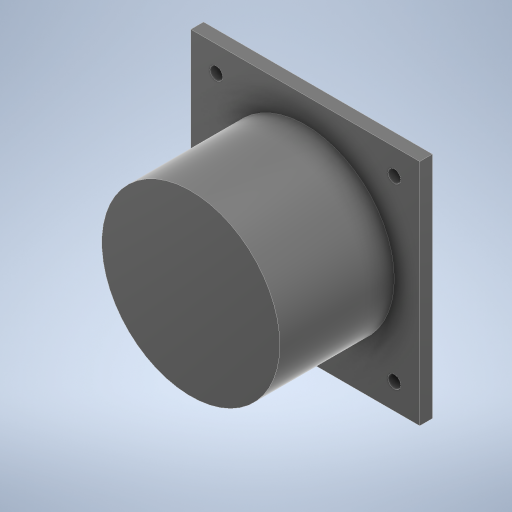
# Autodesk Inventor part: Steckdose
Saved by Autodesk Inventor 2024 (Build 280153000, 153)
## iProperties
Created: 2026-06-01
Part Number: Steckdose
Material: PC/ABS-Kunststoff
Document SubType Name: Modeling
Designer: maxim
Density: 1.1 g/cm^3
Appearance: Glatt - Schwarz
Author: maxim
Autodesk Inventor part; units mm, degrees
ref_plane "YZ Plane" through (0, 0, 0) normal (1, 0, 0) x (0, 1, 0)
ref_plane "XZ Plane" through (0, 0, 0) normal (0, 1, 0) x (-1, 0, 0)
ref_plane "XY Plane" through (0, 0, 0) normal (0, 0, 1) x (1, 0, 0)
sketch "Skizze1" plane through (0, 0, 0) normal (0, 1, 0) x (-1, 0, 0)
  line L0 (0, 0) -> (72, 0)
  line L1 (72, 0) -> (72, -72)
  line L2 (72, -72) -> (0, -72)
  line L3 (0, -72) -> (0, 0)
  dimension "d6" = 72
  dimension "STECKDOSE" = 72
  constraints: 8 end point, 2 parallel, 1 horizontal, 1 perpendicular
  measures "d6" distance of L1.end L2.end
  measures "STECKDOSE" distance of L0.end L1.end
extrude "Extrusion1" add sketch "Skizze1" along normal blind 5
sketch "Skizze2" plane through (0, 5, 0) normal (0, 1, 0) x (1, 0, 0)
  line L0 (-72, 72) -> (-72, 0) projected
  line L1 (0, 0) -> (0, 72) projected
  line L2 (-72, 0) -> (0, 0) projected
  point P0 (-8, 8)
  dimension "d23" = 8
  dimension "d24" = 8
  measures "d23" distance from line of L1 point (-8, 8)
  measures "d24" distance from line of point (-8, 8) L2
hole "Bohrung1" at (-8, 5, -8) direction (0, -1, 0) diameter 4 end through all
pattern_linear "Rechteckige Anordnung1" count 2 spacing 56 along (-1, 0, 0) count 2 spacing 56 along (0, 0, -1) of "Bohrung1"
chamfer "Fasen1" distance 1 angle 45 4 edges at (-36, 5, 0) (-72, 5, -36) (-36, 5, -72) (0, 5, -36)
sketch "Skizze3" plane through (0, 0, 0) normal (0, -1, 0) x (1, 0, 0)
  circle A0 centre (-36, -36) radius 28
  line L0 (-72, 0) -> (0, 0) projected
  line L1 (-72, -72) -> (-72, 0) projected
  point P0 (-36, 0)
  point P1 (-72, -36)
  dimension "d28" = 56
  constraints: 2 midpoint, 1 centre point, 1 horizontal alignment, 1 vertical alignment
  measures "d28" diameter of A0
extrude "Extrusion2" add sketch "Skizze3" along normal blind 36
sketch "Skizze4" plane through (0, 5, 0) normal (0, 1, 0) x (1, 0, 0)
  circle A0 centre (-36, 36) radius 19.5
  line L0 (0, 72) -> (-72, 72) projected
  line L1 (0, 0) -> (0, 72) projected
  point P0 (-36, 72)
  point P1 (0, 36)
  dimension "d31" = 39
  constraints: 2 midpoint, 1 centre point, 1 horizontal alignment, 1 vertical alignment
  measures "d31" diameter of A0
extrude "Extrusion3" cut sketch "Skizze4" against normal blind 28
equation "\"d6\" = STECKDOSE"
